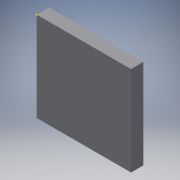
# Autodesk Inventor part: Piso
Saved by Autodesk Inventor 2017 (Build 210142000, 142)
## iProperties
Created: 2021-02-12
Part Number: Piso
Material: Generic
Document SubType Name: Modeling
Designer: USUARIO
Density: 1 g/cm^3
Appearance: Default
Author: USUARIO
Autodesk Inventor part; units mm, degrees
ref_plane "YZ Plane" through (0, 0, 0) normal (1, 0, 0) x (0, 1, 0)
ref_plane "XZ Plane" through (0, 0, 0) normal (0, 1, 0) x (-1, 0, 0)
ref_plane "XY Plane" through (0, 0, 0) normal (0, 0, 1) x (1, 0, 0)
sketch "Sketch1" plane through (0, 0, 0) normal (0, 1, 0) x (-1, 0, 0)
  line L0 (0, 0) -> (390, 0)
  line L1 (390, 0) -> (390, -310)
  line L2 (390, -310) -> (0, -310)
  line L3 (0, -310) -> (0, 0)
  dimension "d0" = 390
  dimension "d1" = 310
  constraints: 8 end point, 2 parallel, 1 horizontal, 1 perpendicular
  measures "d0" distance of L1.end L2.end
  measures "d1" distance of L0.end L1.end
extrude "Extrusion1" add sketch "Sketch1" along normal blind 50.8
body "Solid1"
